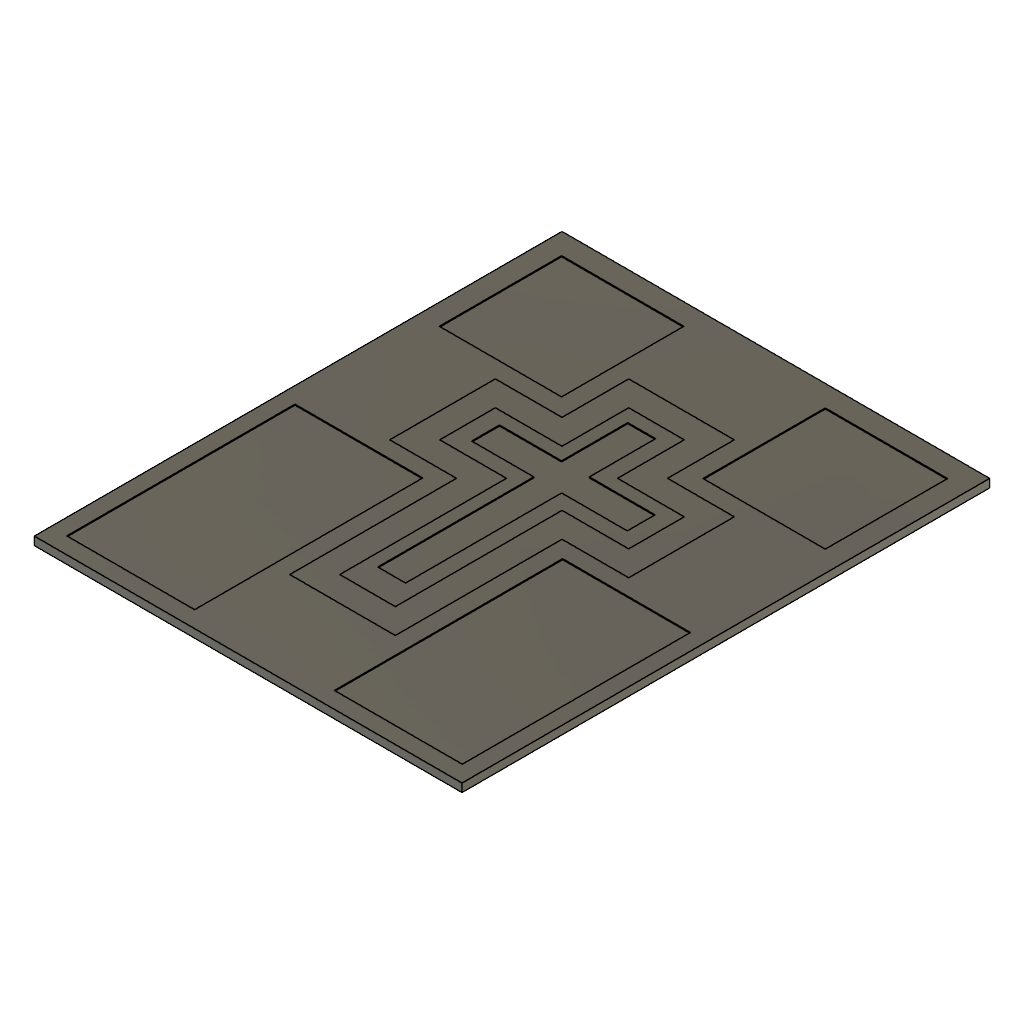
Cross Stencil (Autodesk Fusion 360 design; units mm, degrees)
Autodesk Fusion 360 part; units mm, degrees
sketch "Sketch1" plane through (0, 0, 0) normal (0, 0, 1) x (1, 0, 0)
  line L0 (0, 0) -> (10, 0)
  line L1 (10, 0) -> (10, -12)
  line L2 (10, -12) -> (0, -12)
  line L3 (0, -12) -> (0, 0)
  line L4 (0, -12) -> (-12, -12)
  line L5 (-12, -12) -> (-12, -22)
  line L6 (-12, -22) -> (0, -22)
  line L7 (0, -22) -> (0, -12)
  line L8 (10, -12) -> (22, -12)
  line L9 (22, -12) -> (22, -22)
  line L10 (22, -22) -> (10, -22)
  line L11 (10, -22) -> (10, -12)
  line L12 (0, -22) -> (10, -22)
  line L13 (10, -22) -> (10, -52)
  line L14 (10, -52) -> (0, -52)
  line L15 (0, -52) -> (0, -22)
  dimension "d1" = 10
  dimension "d2" = 12
  dimension "d3" = 12
  dimension "d4" = 10
  dimension "d5" = 12
  dimension "d6" = 10
  dimension "d7" = 30
  constraint horizontal L0
  constraint vertical L1
  constraint horizontal L2
  constraint vertical L3
  constraint coincident L0.start L3.end
  constraint horizontal L4
  constraint vertical L5
  constraint horizontal L6
  constraint vertical L7
  constraint horizontal L8
  constraint vertical L9
  constraint horizontal L10
  constraint vertical L11
  constraint horizontal L12
  constraint vertical L13
  constraint horizontal L14
  constraint vertical L15
  measures "d1" distance of L0.start L0.end
  measures "d2" distance of L0.start L2.end
  measures "d3" distance of L2.end L4.end
  measures "d4" distance of L2.end L6.end
  measures "d5" distance of L1.end L8.end
  measures "d6" distance of L1.end L10.end
  measures "d7" distance of L6.end L14.end
extrude "Extrude1" add sketch "Sketch1" along normal blind 1.5 makes body 1
sketch "Sketch2" plane through (0, 0, 0) normal (0, 0, -1) x (1, 0, 0)
  line L0 (-12, 12) -> (0, 12)
  line L1 (0, 12) -> (0, 0)
  line L2 (0, 0) -> (10, 0)
  line L3 (10, 0) -> (10, 12)
  line L4 (10, 12) -> (22, 12)
  line L5 (22, 12) -> (22, 22)
  line L6 (22, 22) -> (10, 22)
  line L7 (10, 22) -> (10, 52)
  line L8 (10, 52) -> (0, 52)
  line L9 (0, 52) -> (0, 22)
  line L10 (0, 22) -> (-12, 22)
  line L11 (-12, 22) -> (-12, 12)
  line L12 (26.5, 7.5) -> (26.5, 26.5)
  line L13 (26.5, 26.5) -> (14.5, 26.5)
  line L14 (14.5, 26.5) -> (14.5, 56.5)
  line L15 (14.5, 56.5) -> (-4.5, 56.5)
  line L16 (-4.5, 56.5) -> (-4.5, 26.5)
  line L17 (-4.5, 26.5) -> (-16.5, 26.5)
  line L18 (-16.5, 26.5) -> (-16.5, 7.5)
  line L19 (-16.5, 7.5) -> (-4.5, 7.5)
  line L20 (-4.5, 7.5) -> (-4.5, -4.5)
  line L21 (-4.5, -4.5) -> (14.5, -4.5)
  line L22 (14.5, -4.5) -> (14.5, 7.5)
  line L23 (14.5, 7.5) -> (26.5, 7.5)
  line L24 (-4.5, -4.5) -> (-4.5, -21.5)
  line L25 (14.5, 56.5) -> (14.5, 73.5)
  line L26 (14.5, 73.5) -> (43.5, 73.5)
  line L27 (-4.5, -21.5) -> (-33.5, -21.5)
  line L28 (-33.5, -21.5) -> (43.5, -21.5)
  line L29 (43.5, -21.5) -> (43.5, 73.5)
  line L30 (43.5, 73.5) -> (-33.5, 73.5)
  line L31 (-33.5, 73.5) -> (-33.5, -21.5)
  dimension "d10" = 4.5
  dimension "d11" = 17
  dimension "d13" = 17
  dimension "d14" = 29
  dimension "d15" = 29
  constraint perpendicular L21 L24
  constraint perpendicular L15 L25
  constraint perpendicular L25 L26
  constraint perpendicular L24 L27
  constraint horizontal L28
  constraint vertical L29
  constraint horizontal L30
  constraint vertical L31
  measures "d11" distance of L20.end L24.end
  measures "d13" distance of L14.end L25.end
  measures "d14" distance of L25.end L26.end
  measures "d15" distance of L24.end L27.end
extrude "Extrude2" add sketch "Sketch2" against normal blind 1.5 separate body contours L12 L13 L14 L21 L22 L23 L24 L25 L26 L28 L29 L30 | L15 L16 L17 L18 L19 L20 L24 L25 L27 L28 L30 L31 makes body 2
sketch "Sketch3" plane through (0, 0, 1.5) normal (0, 0, 1) x (-1, 0, 0)
  line L0 (-14.5, 7.5) -> (-26.5, 7.5)
  line L1 (-26.5, 7.5) -> (-26.5, 26.5)
  line L2 (-26.5, 26.5) -> (-14.5, 26.5)
  line L3 (-14.5, 26.5) -> (-14.5, 56.5)
  line L4 (-14.5, 56.5) -> (4.5, 56.5)
  line L5 (4.5, 56.5) -> (4.5, 26.5)
  line L6 (4.5, 26.5) -> (16.5, 26.5)
  line L7 (16.5, 26.5) -> (16.5, 7.5)
  line L8 (16.5, 7.5) -> (4.5, 7.5)
  line L9 (4.5, 7.5) -> (4.5, -4.5)
  line L10 (4.5, -4.5) -> (-14.5, -4.5)
  line L11 (-14.5, -4.5) -> (-14.5, 7.5)
  line L12 (33.5, -21.5) -> (33.5, 73.5)
  line L13 (33.5, 73.5) -> (-43.5, 73.5)
  line L14 (-43.5, 73.5) -> (-43.5, -21.5)
  line L15 (-43.5, -21.5) -> (33.5, -21.5)
  line L16 (7.5893, 29.4773) -> (30.5893, 29.4773)
  line L17 (30.5893, 29.4773) -> (30.5893, 70.5409)
  line L18 (30.5893, 70.5409) -> (7.5893, 70.5409)
  line L19 (7.5893, 70.5409) -> (7.5893, 29.4773)
  line L20 (7.732, 4.3436) -> (29.732, 4.3436)
  line L21 (29.732, 4.3436) -> (29.732, -17.6564)
  line L22 (29.732, -17.6564) -> (7.732, -17.6564)
  line L23 (7.732, -17.6564) -> (7.732, 4.3436)
  line L24 (-5, -4.5) -> (-5, -13.4842)
  line L25 (8.9329, 14.3198) -> (-19.0671, 14.3198)
  line L26 (-19.0671, 14.3198) -> (-19.0671, 19.3198)
  line L27 (-19.0671, 19.3198) -> (8.9329, 19.3198)
  line L28 (8.9329, 19.3198) -> (8.9329, 14.3198)
  line L29 (-2.2442, 2.4038) -> (-7.2442, 2.4038)
  line L30 (-7.2442, 2.4038) -> (-7.2442, 47.4038)
  line L31 (-7.2442, 47.4038) -> (-2.2442, 47.4038)
  line L32 (-2.2442, 47.4038) -> (-2.2442, 2.4038)
  line L33 (-17.732, 4.3436) -> (-39.732, 4.3436)
  line L34 (-39.732, 4.3436) -> (-39.732, -17.6564)
  line L35 (-39.732, -17.6564) -> (-17.732, -17.6564)
  line L36 (-17.732, -17.6564) -> (-17.732, 4.3436)
  line L37 (-17.5893, 29.4773) -> (-40.5893, 29.4773)
  line L38 (-17.5893, 70.5409) -> (-17.5893, 29.4773)
  line L39 (-40.5893, 29.4773) -> (-40.5893, 70.5409)
  line L40 (-40.5893, 70.5409) -> (-17.5893, 70.5409)
  dimension "d18" = 23
  dimension "d19" = 22
  dimension "d20" = 22
  dimension "d21" = 28
  dimension "d22" = 5
  dimension "d23" = 5
  dimension "d24" = 45
  constraint horizontal L16
  constraint vertical L17
  constraint horizontal L18
  constraint vertical L19
  constraint horizontal L20
  constraint vertical L21
  constraint horizontal L22
  constraint vertical L23
  constraint midpoint L10 L24.start
  constraint perpendicular L10 L24
  constraint horizontal L25
  constraint vertical L26
  constraint horizontal L27
  constraint vertical L28
  constraint horizontal L29
  constraint vertical L30
  constraint horizontal L31
  constraint vertical L32
  constraint symmetric L16.start L24 L37.start
  constraint symmetric L16.end L24 L37.end
  constraint symmetric L17.end L24 L39.end
  constraint symmetric L18.end L24 L38.start
  constraint symmetric L20.start L24 L33.start
  constraint symmetric L20.end L24 L33.end
  constraint symmetric L21.end L24 L34.end
  constraint symmetric L22.end L24 L35.end
  measures "d18" distance of L16.start L16.end
  measures "d19" distance of L20.start L20.end
  measures "d20" distance of L20.start L22.end
  measures "d21" distance of L25.start L25.end
  measures "d22" distance of L25.start L27.end
  measures "d23" distance of L29.start L29.end
  measures "d24" distance of L29.start L31.end
extrude "Extrude3" cut sketch "Sketch3" against normal blind 0.15 contours L16 L17 L18 L19 | L20 L21 L22 L23 | L25 L27 L28 L32 | L25 L29 L30 L32 | L25 L27 L30 L32 | L25 L26 L27 L30 | L27 L30 L31 L32 | L33 L34 L35 L36 | L37 L38 L39 L40 bodies 1 2
sketch "Sketch4" plane through (0, 0, 0) normal (0, 0, 1) x (1, 0, 0)
  line L0 (0, -12) -> (-12, -12)
  line L1 (0, 0) -> (0, -12)
  line L2 (10, 0) -> (0, 0)
  line L3 (7.2442, -19.3198) -> (7.2442, -47.4038)
  line L4 (7.2442, -47.4038) -> (2.2442, -47.4038)
  line L5 (2.2442, -47.4038) -> (2.2442, -19.3198)
  line L6 (2.2442, -19.3198) -> (-8.9329, -19.3198)
  line L7 (-8.9329, -19.3198) -> (-8.9329, -14.3198)
  line L8 (-8.9329, -14.3198) -> (2.2442, -14.3198)
  line L9 (2.2442, -14.3198) -> (2.2442, -2.4038)
  line L10 (2.2442, -2.4038) -> (7.2442, -2.4038)
  line L11 (7.2442, -2.4038) -> (7.2442, -14.3198)
  line L12 (7.2442, -14.3198) -> (19.0671, -14.3198)
  line L13 (19.0671, -14.3198) -> (19.0671, -19.3198)
  line L14 (19.0671, -19.3198) -> (7.2442, -19.3198)
  line L15 (0, -12) -> (-12, -12)
  line L16 (-12, -12) -> (-12, -22)
  line L17 (-12, -22) -> (0, -22)
  line L18 (0, -22) -> (0, -52)
  line L19 (0, -52) -> (10, -52)
  line L20 (10, -52) -> (10, -22)
  line L21 (10, -22) -> (22, -22)
  line L22 (22, -22) -> (22, -12)
  line L23 (22, -12) -> (10, -12)
  line L24 (10, -12) -> (10, 0)
  line L25 (10, 0) -> (0, 0)
  line L26 (0, 0) -> (0, -12)
  line L27 (39.732, -4.3436) -> (17.732, -4.3436)
  line L28 (17.732, -4.3436) -> (17.732, 17.6564)
  line L29 (17.732, 17.6564) -> (39.732, 17.6564)
  line L30 (39.732, 17.6564) -> (39.732, -4.3436)
  line L31 (-30.5893, -29.4773) -> (-7.5893, -29.4773)
  line L32 (-7.5893, -29.4773) -> (-7.5893, -70.5409)
  line L33 (-7.5893, -70.5409) -> (-30.5893, -70.5409)
  line L34 (-30.5893, -70.5409) -> (-30.5893, -29.4773)
  line L35 (-29.732, -4.3436) -> (-29.732, 17.6564)
  line L36 (-29.732, 17.6564) -> (-7.732, 17.6564)
  line L37 (-7.732, 17.6564) -> (-7.732, -4.3436)
  line L38 (-7.732, -4.3436) -> (-29.732, -4.3436)
  line L39 (17.5893, -29.4773) -> (40.5893, -29.4773)
  line L40 (40.5893, -29.4773) -> (40.5893, -70.5409)
  line L41 (40.5893, -70.5409) -> (17.5893, -70.5409)
  line L42 (17.5893, -70.5409) -> (17.5893, -29.4773)
  line L43 (14.5, -7.5) -> (26.5, -7.5)
  line L44 (26.5, -7.5) -> (26.5, -26.5)
  line L45 (26.5, -26.5) -> (14.5, -26.5)
  line L46 (14.5, -26.5) -> (14.5, -56.5)
  line L47 (14.5, -56.5) -> (-4.5, -56.5)
  line L48 (-4.5, -56.5) -> (-4.5, -26.5)
  line L49 (-4.5, -26.5) -> (-16.5, -26.5)
  line L50 (-16.5, -26.5) -> (-16.5, -7.5)
  line L51 (-16.5, -7.5) -> (-4.5, -7.5)
  line L52 (-4.5, -7.5) -> (-4.5, 4.5)
  line L53 (-4.5, 4.5) -> (14.5, 4.5)
  line L54 (14.5, 4.5) -> (14.5, -7.5)
  line L55 (-33.5, 21.5) -> (-33.5, -73.5)
  line L56 (-33.5, -73.5) -> (43.5, -73.5)
  line L57 (43.5, -73.5) -> (43.5, 21.5)
  line L58 (43.5, 21.5) -> (-33.5, 21.5)
extrude "Extrude4" add sketch "Sketch4" along normal blind 1.5 separate body contours L43 L44 L45 L46 L47 L48 L49 L50 L51 L52 L53 L54 makes body 3
equation "d13 = d11"
equation "d14 = d13 + 12 mm"
equation "d15 = d11 + 12 mm"
